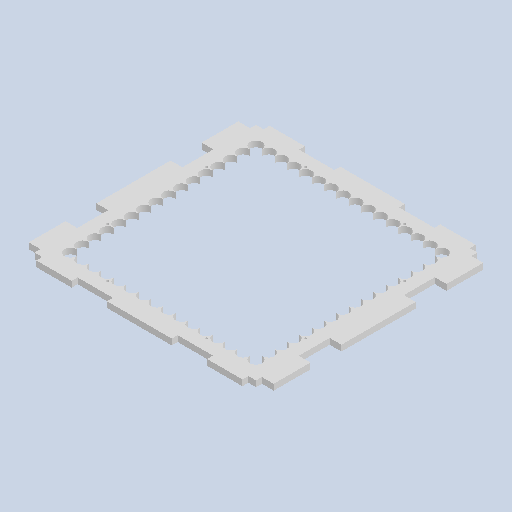
# Autodesk Inventor part: NewBoardHolder
Saved by Autodesk Inventor 2022 (Build 260153000, 153)
## iProperties
Created: 2021-06-29
Part Number: NewBoardHolder
Material: Generic
Document SubType Name: Modeling
Designer: benka
Density: 1 g/cm^3
Appearance: Default
Author: benka
Autodesk Inventor part; units mm, degrees
ref_plane "YZ Plane" through (0, 0, 0) normal (1, 0, 0) x (0, 1, 0)
ref_plane "XZ Plane" through (0, 0, 0) normal (0, 1, 0) x (-1, 0, 0)
ref_plane "XY Plane" through (0, 0, 0) normal (0, 0, 1) x (1, 0, 0)
sketch "Sketch3" plane through (-0.0872, 0, 0.1488) normal (0, 1, 0) x (-1, 0, 0)
  circle A0 centre (-84.0872, -42.1488) radius 1
  line L0 (-94.0872, -57.8988) -> (-94.0872, -31.6488)
  line L1 (-27.5872, -94.1488) -> (-27.5872, -99.1488)
  line L2 (-27.5872, -99.1488) -> (27.4128, -99.1488)
  line L3 (27.4128, -94.1488) -> (27.4128, -99.1488)
  circle A1 centre (-42.0872, -84.1488) radius 1
  line L4 (-57.5872, -94.1488) -> (-27.5872, -94.1488)
  line L5 (-57.5872, -94.1488) -> (-57.5872, -99.1488)
  line L6 (-87.5872, -99.1488) -> (-57.5872, -99.1488)
  line L7 (-104.0872, -57.8988) -> (-104.0872, -89.1488)
  line L8 (-104.0872, -57.8988) -> (-94.0872, -57.8988)
  line L9 (-94.0872, -89.1488) -> (-104.0872, -89.1488)
  line L10 (-94.0872, -89.1488) -> (-94.0872, -94.1488)
  line L11 (-94.0872, -94.1488) -> (-87.5872, -94.1488)
  line L12 (-87.5872, -94.1488) -> (-87.5872, -99.1488)
  line L13 (-104.0872, 31.3512) -> (-104.0872, -31.6488)
  line L14 (-104.0872, -31.6488) -> (-94.0872, -31.6488)
  circle A2 centre (-84.0872, 41.8512) radius 1
  line L15 (-94.0872, 31.3512) -> (-94.0872, 57.6012)
  line L16 (-104.0872, 31.3512) -> (-94.0872, 31.3512)
  line L17 (-104.0872, 57.6012) -> (-94.0872, 57.6012)
  line L18 (-94.0872, 88.8512) -> (-104.0872, 88.8512)
  line L19 (-104.0872, 88.8512) -> (-104.0872, 57.6012)
  circle A3 centre (-42.0872, 83.8512) radius 1
  line L20 (-87.5872, 98.8512) -> (-87.5872, 93.8512)
  line L21 (-94.0872, 93.8512) -> (-87.5872, 93.8512)
  line L22 (-94.0872, 88.8512) -> (-94.0872, 93.8512)
  line L23 (-87.5872, 98.8512) -> (-57.5872, 98.8512)
  line L24 (-57.5872, 93.8512) -> (-57.5872, 98.8512)
  line L25 (-57.5872, 93.8512) -> (-27.5872, 93.8512)
  line L26 (-27.5872, 93.8512) -> (-27.5872, 98.8512)
  line L27 (-27.5872, 98.8512) -> (27.4128, 98.8512)
  line L28 (27.4128, 93.8512) -> (27.4128, 98.8512)
  circle A4 centre (41.9128, -84.1488) radius 1
  line L29 (93.9128, -57.8988) -> (93.9128, -31.6488)
  circle A5 centre (83.9128, -42.1488) radius 1
  line L30 (103.9128, -57.8988) -> (93.9128, -57.8988)
  line L31 (103.9128, -89.1488) -> (103.9128, -57.8988)
  line L32 (103.9128, -89.1488) -> (93.9128, -89.1488)
  line L33 (57.4128, -94.1488) -> (57.4128, -99.1488)
  line L34 (57.4128, -99.1488) -> (87.4128, -99.1488)
  line L35 (87.4128, -94.1488) -> (87.4128, -99.1488)
  line L36 (93.9128, -94.1488) -> (87.4128, -94.1488)
  line L37 (93.9128, -89.1488) -> (93.9128, -94.1488)
  line L38 (103.9128, -31.6488) -> (93.9128, -31.6488)
  line L39 (27.4128, -94.1488) -> (57.4128, -94.1488)
  line L40 (103.9128, 31.3512) -> (93.9128, 31.3512)
  line L41 (103.9128, 57.6012) -> (93.9128, 57.6012)
  line L42 (103.9128, 57.6012) -> (103.9128, 88.8512)
  line L43 (93.9128, 93.8512) -> (87.4128, 93.8512)
  line L44 (93.9128, 88.8512) -> (103.9128, 88.8512)
  line L45 (93.9128, 88.8512) -> (93.9128, 93.8512)
  line L46 (27.4128, 93.8512) -> (57.4128, 93.8512)
  circle A6 centre (41.9128, 83.8512) radius 1
  circle A7 centre (83.9128, 41.8512) radius 1
  line L47 (57.4128, 93.8512) -> (57.4128, 98.8512)
  line L48 (93.9128, 31.3512) -> (93.9128, 57.6012)
  line L49 (57.4128, 98.8512) -> (87.4128, 98.8512)
  line L50 (87.4128, 93.8512) -> (87.4128, 98.8512)
  line L51 (103.9128, -31.6488) -> (103.9128, 31.3512)
  arc A8 (-73.5872, 78.6012) -> (-78.8372, 73.3512) centre (-78.8372, 78.6012) ccw
  arc A9 (-63.0872, 78.6012) -> (-73.5872, 78.6012) centre (-68.3372, 78.6012) ccw
  arc A10 (-78.8372, 73.3512) -> (-78.8372, 62.8512) centre (-78.8372, 68.1012) ccw
  arc A11 (-52.5872, 78.6012) -> (-63.0872, 78.6012) centre (-57.8372, 78.6012) ccw
  arc A12 (-42.0872, 78.6012) -> (-52.5872, 78.6012) centre (-47.3372, 78.6012) ccw
  arc A13 (-31.5872, 78.6012) -> (-42.0872, 78.6012) centre (-36.8372, 78.6012) ccw
  arc A14 (-21.0872, 78.6012) -> (-31.5872, 78.6012) centre (-26.3372, 78.6012) ccw
  arc A15 (-10.5872, 78.6012) -> (-21.0872, 78.6012) centre (-15.8372, 78.6012) ccw
  arc A16 (-0.0872, 78.6012) -> (-10.5872, 78.6012) centre (-5.3372, 78.6012) ccw
  arc A17 (10.4128, 78.6012) -> (-0.0872, 78.6012) centre (5.1628, 78.6012) ccw
  arc A18 (20.9128, 78.6012) -> (10.4128, 78.6012) centre (15.6628, 78.6012) ccw
  arc A19 (31.4128, 78.6012) -> (20.9128, 78.6012) centre (26.1628, 78.6012) ccw
  arc A20 (41.9128, 78.6012) -> (31.4128, 78.6012) centre (36.6628, 78.6012) ccw
  arc A21 (52.4128, 78.6012) -> (41.9128, 78.6012) centre (47.1628, 78.6012) ccw
  arc A22 (62.9128, 78.6012) -> (52.4128, 78.6012) centre (57.6628, 78.6012) ccw
  arc A23 (73.4128, 78.6012) -> (62.9128, 78.6012) centre (68.1628, 78.6012) ccw
  arc A24 (-78.8372, 62.8512) -> (-78.8372, 52.3512) centre (-78.8372, 57.6012) ccw
  arc A25 (-78.8372, 52.3512) -> (-78.8372, 41.8512) centre (-78.8372, 47.1012) ccw
  arc A26 (-78.8372, 41.8512) -> (-78.8372, 31.3512) centre (-78.8372, 36.6012) ccw
  arc A27 (-78.8372, 31.3512) -> (-78.8372, 20.8512) centre (-78.8372, 26.1012) ccw
  arc A28 (-78.8372, 20.8512) -> (-78.8372, 10.3512) centre (-78.8372, 15.6012) ccw
  arc A29 (-78.8372, 10.3512) -> (-78.8372, -0.1488) centre (-78.8372, 5.1012) ccw
  arc A30 (78.6628, -0.1488) -> (78.6628, 10.3512) centre (78.6628, 5.1012) ccw
  arc A31 (78.6628, 10.3512) -> (78.6628, 20.8512) centre (78.6628, 15.6012) ccw
  arc A32 (78.6628, 20.8512) -> (78.6628, 31.3512) centre (78.6628, 26.1012) ccw
  arc A33 (78.6628, 31.3512) -> (78.6628, 41.8512) centre (78.6628, 36.6012) ccw
  arc A34 (78.6628, 73.3512) -> (73.4128, 78.6012) centre (78.6628, 78.6012) ccw
  arc A35 (78.6628, 62.8512) -> (78.6628, 73.3512) centre (78.6628, 68.1012) ccw
  arc A36 (78.6628, 52.3512) -> (78.6628, 62.8512) centre (78.6628, 57.6012) ccw
  arc A37 (78.6628, 41.8512) -> (78.6628, 52.3512) centre (78.6628, 47.1012) ccw
  arc A38 (-78.8372, -73.6488) -> (-73.5872, -78.8988) centre (-78.8372, -78.8988) ccw
  arc A39 (-73.5872, -78.8988) -> (-63.0872, -78.8988) centre (-68.3372, -78.8988) ccw
  arc A40 (78.6628, -10.6488) -> (78.6628, -0.1488) centre (78.6628, -5.3988) ccw
  arc A41 (78.6628, -21.1488) -> (78.6628, -10.6488) centre (78.6628, -15.8988) ccw
  arc A42 (78.6628, -31.6488) -> (78.6628, -21.1488) centre (78.6628, -26.3988) ccw
  arc A43 (78.6628, -42.1488) -> (78.6628, -31.6488) centre (78.6628, -36.8988) ccw
  arc A44 (31.4128, -78.8988) -> (41.9128, -78.8988) centre (36.6628, -78.8988) ccw
  arc A45 (-10.5872, -78.8988) -> (-0.0872, -78.8988) centre (-5.3372, -78.8988) ccw
  arc A46 (-0.0872, -78.8988) -> (10.4128, -78.8988) centre (5.1628, -78.8988) ccw
  arc A47 (10.4128, -78.8988) -> (20.9128, -78.8988) centre (15.6628, -78.8988) ccw
  arc A48 (20.9128, -78.8988) -> (31.4128, -78.8988) centre (26.1628, -78.8988) ccw
  arc A49 (-63.0872, -78.8988) -> (-52.5872, -78.8988) centre (-57.8372, -78.8988) ccw
  arc A50 (-21.0872, -78.8988) -> (-10.5872, -78.8988) centre (-15.8372, -78.8988) ccw
  arc A51 (-31.5872, -78.8988) -> (-21.0872, -78.8988) centre (-26.3372, -78.8988) ccw
  arc A52 (-42.0872, -78.8988) -> (-31.5872, -78.8988) centre (-36.8372, -78.8988) ccw
  arc A53 (-52.5872, -78.8988) -> (-42.0872, -78.8988) centre (-47.3372, -78.8988) ccw
  arc A54 (41.9128, -78.8988) -> (52.4128, -78.8988) centre (47.1628, -78.8988) ccw
  arc A55 (52.4128, -78.8988) -> (62.9128, -78.8988) centre (57.6628, -78.8988) ccw
  arc A56 (62.9128, -78.8988) -> (73.4128, -78.8988) centre (68.1628, -78.8988) ccw
  arc A57 (78.6628, -52.6488) -> (78.6628, -42.1488) centre (78.6628, -47.3988) ccw
  arc A58 (78.6628, -63.1488) -> (78.6628, -52.6488) centre (78.6628, -57.8988) ccw
  arc A59 (78.6628, -73.6488) -> (78.6628, -63.1488) centre (78.6628, -68.3988) ccw
  arc A60 (73.4128, -78.8988) -> (78.6628, -73.6488) centre (78.6628, -78.8988) ccw
  arc A61 (-78.8372, -21.1488) -> (-78.8372, -31.6488) centre (-78.8372, -26.3988) ccw
  arc A62 (-78.8372, -31.6488) -> (-78.8372, -42.1488) centre (-78.8372, -36.8988) ccw
  arc A63 (-78.8372, -42.1488) -> (-78.8372, -52.6488) centre (-78.8372, -47.3988) ccw
  arc A64 (-78.8372, -10.6488) -> (-78.8372, -21.1488) centre (-78.8372, -15.8988) ccw
  arc A65 (-78.8372, -0.1488) -> (-78.8372, -10.6488) centre (-78.8372, -5.3988) ccw
  arc A66 (-78.8372, -63.1488) -> (-78.8372, -73.6488) centre (-78.8372, -68.3988) ccw
  arc A67 (-78.8372, -52.6488) -> (-78.8372, -63.1488) centre (-78.8372, -57.8988) ccw
  point P0 (-104.0094, 88.5791)
  point P1 (-0.0872, -0.1488)
  point P2 (-0.0001, 0)
  dimension "d154" = 31.25
  dimension "d175" = 2
  dimension "d177" = 2
  dimension "d165" = 2
  dimension "d161" = 2
  dimension "d149" = 2
  dimension "d158" = 2
  dimension "d150" = 84
  dimension "d166" = 84
  dimension "d151" = 84
  dimension "d155" = 30
  dimension "d156" = 30
  dimension "d176" = 55
  dimension "d174" = 30
  dimension "d169" = 30
  dimension "d172" = 10
  dimension "d171" = 5
  dimension "d173" = 31.25
  dimension "d167" = 26.25
  dimension "d164" = 63
  dimension "d163" = 26.25
  dimension "d162" = 31.25
  dimension "d160" = 5
  dimension "d159" = 5
  dimension "d170" = 5
  dimension "d168" = 6.5
  dimension "d181" = 5
  dimension "d157" = 31.25
  dimension "d182" = 26.25
  dimension "d183" = 63
  dimension "d184" = 26.25
  dimension "d152" = 5
  dimension "d147" = 5
  dimension "d153" = 10
  dimension "d185" = 6.5
  dimension "d186" = 30
  dimension "d187" = 55
  dimension "d188" = 30
  dimension "d189" = 30
  dimension "d190" = 6.5
  dimension "d191" = 10
  dimension "d148" = 5
  dimension "d192" = 5
  dimension "d146" = 104
  dimension "d145" = 99
  dimension "d144" = 84
  dimension "d143" = 84
  dimension "d142" = 84
  dimension "d141" = 84
  dimension "d140" = 42
  dimension "d139" = 42
  dimension "d193" = 42
  dimension "d194" = 42
  dimension "d138" = 84
  dimension "d137" = 42
  dimension "d195" = 42
  dimension "d136" = 42
  dimension "d196" = 42
  dimension "d135" = 84
  dimension "d134" = 84
  dimension "d125" = 10.5
  dimension "d119" = 10.5
  dimension "d131" = 15.25
  dimension "d130" = 15.25
  constraints: 120 point on circle, 105 end point, 68 centre point, 49 perpendicular, 25 collinear, 2 vertical, 1 horizontal, 1 other
  measures "d154" distance of L42.end L41.start
  measures "d175" diameter of A1
  measures "d177" diameter of A0
  measures "d165" diameter of A2
  measures "d161" diameter of A3
  measures "d149" diameter of A7
  measures "d158" diameter of A5
  measures "d150" distance of A5.centre A7.centre
  measures "d166" distance of A2.centre A0.centre
  measures "d151" distance of A3.centre A6.centre
  measures "d155" distance between parallel lines of L33 L35
  measures "d156" distance between parallel lines of L3 L33
  measures "d176" distance between parallel lines of L1 L3
  measures "d174" distance between parallel lines of L5 L1
  measures "d169" distance between parallel lines of L12 L5
  measures "d172" distance between parallel lines of L7 L10
  measures "d171" distance between parallel lines of L9 L11
  measures "d173" distance between parallel lines of L8 L9
  measures "d167" distance between parallel lines of L14 L8
  measures "d164" distance between parallel lines of L16 L14
  measures "d163" distance between parallel lines of L17 L16
  measures "d162" distance between parallel lines of L18 L17
  measures "d160" distance between parallel lines of L18 L21
  measures "d159" distance between parallel lines of L23 L21
  measures "d170" distance between parallel lines of L6 L11
  measures "d168" distance between parallel lines of L10 L12
  measures "d181" distance between parallel lines of L36 L34
  measures "d157" distance of L31.start L30.start
  measures "d182" distance of L29.start L29.end
  measures "d183" distance of L38.start L40.start
  measures "d184" distance of L40.end L41.end
  measures "d152" distance of L44.start L43.start
  measures "d147" distance of L43.end L49.end
  measures "d153" distance of L44.start L42.end
  measures "d185" distance of L43.start L43.end
  measures "d186" distance of L47.end L49.end
  measures "d187" distance of L26.end L27.end
  measures "d188" distance of L24.start L25.end
  measures "d189" distance of L20.start L23.end
  measures "d190" distance of L21.start L20.end
  measures "d191" distance of L18.start L18.end
  measures "d148" distance of L46.end L47.end
  measures "d192" distance of L28.start L27.end
  measures "d146" distance from line of L51 point (-0.087, -0.149)
  measures "d145" distance from line of L27 point (-0.087, -0.149)
  measures "d144" horizontal distance of A5.centre point (-0.087, -0.149)
  measures "d143" horizontal distance of A0.centre point (-0.087, -0.149)
  measures "d142" horizontal distance of A7.centre point (-0.087, -0.149)
  measures "d141" horizontal distance of A2.centre point (-0.087, -0.149)
  measures "d140" vertical distance of A2.centre point (-0.087, -0.149)
  measures "d139" vertical distance of A7.centre point (-0.087, -0.149)
  measures "d193" vertical distance of A5.centre point (-0.087, -0.149)
  measures "d194" vertical distance of A0.centre point (-0.087, -0.149)
  measures "d138" vertical distance of A1.centre point (-0.087, -0.149)
  measures "d137" horizontal distance of A4.centre point (-0.087, -0.149)
  measures "d195" horizontal distance of A1.centre point (-0.087, -0.149)
  measures "d136" horizontal distance of A6.centre point (-0.087, -0.149)
  measures "d196" horizontal distance of A3.centre point (-0.087, -0.149)
  measures "d135" vertical distance of A6.centre point (-0.087, -0.149)
  measures "d134" vertical distance of A3.centre point (-0.087, -0.149)
  measures "d125" distance of A9.centre A11.centre
  measures "d119" distance of A10.centre A24.centre
  measures "d131" distance from line of L0 A63.centre
  measures "d130" distance from line of L29 A57.centre
extrude "newBoardHolder" add sketch "Sketch3" along normal blind 5
body "Solid1"
